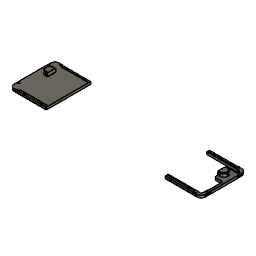
Pianista_podpera_klasvesy (Autodesk Fusion 360 design; units mm, degrees)
Autodesk Fusion 360 part; units mm, degrees
note: some values were not read from the file. Chosen so that the rebuilt part matches the saved one: which face or edge a step refers to. Set by a fixed rule: which sketch regions a step uses.
sketch "Sketch1" plane through (0, 0, 0) normal (0, 0, 1) x (1, 0, 0)
  line L0 (0, 0) -> (-465, 0)
  line L1 (-465, 0) -> (-465, 250)
  line L2 (-465, 250) -> (0, 250)
  line L3 (-275, 250) -> (-275, 0)
  line L4 (0, 0) -> (465, 0)
  line L5 (465, 0) -> (465, 250)
  line L6 (275, 250) -> (275, 0)
  line L7 (465, 250) -> (0, 250)
  line L8 (0, 0) -> (0, 110)
  line L9 (-443, 13) -> (-443, 222)
  line L10 (-443, 222) -> (0, 222)
  line L11 (443, 13) -> (443, 222)
  line L12 (443, 222) -> (0, 222)
  line L13 (0, 13) -> (443, 13)
  line L14 (0, 13) -> (-443, 13)
  line L15 (-465, 250) -> (-465, 176.5)
  line L16 (-465, 0) -> (-465, 145.5)
  line L17 (-422.875, 157.5) -> (-422.875, 176.5)
  line L18 (-423, 157.5) -> (-423, 138.5)
  line L19 (-465, 0) -> (-438, 0)
  circle A0 centre (-438, 45) radius 3
  circle A1 centre (438, 45) radius 3
  circle A2 centre (-438, 45) radius 1.8
  circle A3 centre (438, 45) radius 1.8
  line L20 (0, 28) -> (-425, 28)
  line L21 (-423, 207) -> (0, 207)
  line L22 (-398.9602, 123.8181) -> (-428.0977, 123.2487)
  line L23 (-394.0579, 128.8187) -> (-394.075, 186.5015)
  line L24 (-399.075, 191.5) -> (-428, 191.5)
  line L25 (-430, 33) -> (-430, 55)
  line L26 (-433, 57) -> (-433, 118.2497)
  arc A4 (-423, 207) -> (-433, 197) centre (-423, 197) ccw
  arc A5 (-430, 33) -> (-425, 28) centre (-425, 33) ccw
  arc A6 (-394.075, 186.5015) -> (-399.075, 191.5) centre (-399.075, 186.5) ccw
  arc A7 (-398.9602, 123.8181) -> (-394.0579, 128.8187) centre (-399.0579, 128.8172) ccw
  arc A8 (-428.0977, 123.2487) -> (-433, 118.2497) centre (-428, 118.2497) ccw
  line L27 (-433, 197) -> (-433, 196.5)
  arc A9 (-433, 196.5) -> (-428, 191.5) centre (-428, 196.5) ccw
  line L28 (-404.0722, 177) -> (-275, 177)
  line L29 (-404.075, 138.4) -> (-275, 138.4)
  line L30 (423, 207) -> (0, 207)
  arc A10 (433, 197) -> (423, 207) centre (423, 197) ccw
  line L31 (433, 197) -> (433, 196.5)
  arc A11 (428, 191.5) -> (433, 196.5) centre (428, 196.5) ccw
  line L32 (399.075, 191.5) -> (428, 191.5)
  line L33 (404.0722, 177) -> (275, 177)
  line L34 (404.075, 138.4) -> (275, 138.4)
  line L35 (394.0579, 128.8187) -> (394.075, 186.5015)
  arc A12 (399.075, 191.5) -> (394.075, 186.5015) centre (399.075, 186.5) ccw
  line L36 (-432, 56) -> (-431, 56)
  arc A13 (-433, 57) -> (-432, 56) centre (-432, 57) ccw
  arc A14 (-430, 55) -> (-431, 56) centre (-431, 55) ccw
  arc A15 (394.0579, 128.8187) -> (398.9602, 123.8181) centre (399.0579, 128.8172) ccw
  line L37 (398.9602, 123.8181) -> (428.0977, 123.2487)
  arc A16 (433, 118.2497) -> (428.0977, 123.2487) centre (428, 118.2497) ccw
  line L38 (433, 57) -> (433, 118.2497)
  arc A17 (432, 56) -> (433, 57) centre (432, 57) ccw
  line L39 (432, 56) -> (431, 56)
  arc A18 (431, 56) -> (430, 55) centre (431, 55) ccw
  line L40 (430, 33) -> (430, 55)
  arc A19 (425, 28) -> (430, 33) centre (425, 33) ccw
  line L41 (0, 28) -> (425, 28)
  arc A20 (-404.0722, 177) -> (-404.075, 138.4) centre (-403.6974, 157.7) ccw
  arc A21 (404.075, 138.4) -> (404.0722, 177) centre (403.6974, 157.7) ccw
  point P0 (-394.0765, 191.5)
  dimension "d1" = 465
  dimension "d2" = 250
  dimension "d33" = 550
  dimension "d96" = 73.5
  dimension "d97" = 145.5
  dimension "d104" = 19
  dimension "d105" = 42
  dimension "d114" = 27
  dimension "d115" = 45
  dimension "d116" = 6
  dimension "d120" = 3.6
  dimension "d127" = 15
  dimension "d128" = 15
  dimension "d129" = 10
  dimension "d131" = 5
  dimension "d132" = 5
  dimension "d133" = 5
  dimension "d134" = 5
  dimension "d135" = 5
  dimension "d138" = 10
  dimension "d139" = 14.5
  dimension "d144" = 38.6
  dimension "d145" = 1
  dimension "d146" = 1
  constraint coincident L0.start L4.start
  constraint perpendicular L0 L8
  constraint perpendicular L0 L1
  constraint perpendicular L0 L3
  constraint symmetric L0.start L4.start L8
  constraint symmetric L0.end L4.end L8
  constraint symmetric L1.end L5.end L8
  constraint coincident L2 L3.start
  constraint coincident L0 L3.end
  constraint perpendicular L2 L15
  constraint perpendicular L0 L16
  constraint perpendicular L16 L19
  constraint symmetric L8 A0 A1
  constraint concentric A0 A2
  constraint symmetric L8 A2 A3
  constraint perpendicular L9 L24
  constraint coincident P0 L23
  constraint tangent L21 A4
  constraint tangent L26 A4
  constraint tangent L25 A5
  constraint tangent L20 A5
  constraint coincident P0 L24
  constraint tangent L24 A6
  constraint tangent L23 A6
  constraint tangent L22 A7
  constraint tangent L23 A7
  constraint coincident L26 A4.end
  constraint tangent L26 A8
  constraint tangent L22 A8
  constraint tangent A4 L27
  constraint perpendicular L24 L27
  constraint tangent L27 A9
  constraint tangent L24 A9
  constraint coincident L18.start A20
  constraint symmetric L8 L21.end L30.end
  constraint symmetric L8 L21.start L30.start
  constraint symmetric L8 A4.end A10.start
  constraint symmetric L8 A4 A10
  constraint symmetric L8 L24.start L32.start
  constraint symmetric L8 L23.end L35.end
  constraint symmetric L8 A6 A12
  constraint symmetric L8 L23.start L35.start
  constraint symmetric L8 L27.end L31.end
  constraint symmetric L8 L24.end A11.start
  constraint symmetric L8 A9 A11
  constraint symmetric L8 L28.start L33.start
  constraint symmetric L8 L28.end L33.end
  constraint symmetric L8 L29.start L34.start
  constraint symmetric L8 L29.end L34.end
  constraint symmetric L8 A20 A21
  constraint perpendicular L25 L36
  constraint tangent L26 A13
  constraint tangent L36 A13
  constraint tangent L36 A14
  constraint tangent L25 A14
  constraint symmetric L8 L20.start L41.start
  constraint symmetric L8 L25.start L40.start
  constraint symmetric L8 L20.end A19.start
  constraint symmetric L8 A5 A19
  constraint symmetric L8 L22.start A15.end
  constraint symmetric L8 A7 A15
  constraint symmetric L8 L26.end A16.start
  constraint symmetric L8 L22.end L37.end
  constraint symmetric L8 A8 A16
  constraint symmetric L8 L26.start L38.start
  constraint symmetric L8 L36.start A17.start
  constraint symmetric L8 A13 A17
  constraint symmetric L8 L36.end L39.end
  constraint symmetric L8 L25.end A18.end
  constraint symmetric L8 A14 A18
  measures "d1" distance of L0.start L0.end
  measures "d2" distance of L0.start L2.end
  measures "d33" distance of L3.end L6.end
  measures "d96" distance of L1.end L15.end
  measures "d97" distance of L0.end L16.end
  measures "d104" distance of L17.start L17.end
  measures "d105" distance of L1 L18.start
  measures "d114" distance of L0.end L19.end
  measures "d115" distance of L19.end A0.centre
  measures "d116" diameter of A0
  measures "d120" diameter of A2
  measures "d127" distance of L10 L21
  measures "d128" distance of L14 L20
  measures "d129" radius of A4
  measures "d131" radius of A5
  measures "d132" radius of A6
  measures "d133" radius of A7
  measures "d134" radius of A8
  measures "d135" radius of A9
  measures "d138" distance of L23 L28.start
  measures "d139" distance of L24 L28.start
  measures "d144" distance of L28 L29
  measures "d145" radius of A13
  measures "d146" radius of A14
extrude "Extrude1" add sketch "Sketch1" along normal blind 11.5 contours L3 L9 L10 L14 L20 L21 L22 L23 L24 L25 L26 A4 A5 A6 A7 A8 L27 A9 L28 L29 L36 A13 A14 A20 | L6 L11 L12 L13 L30 A10 L31 A11 L32 L33 L34 L35 A12 A15 L37 A16 L38 A17 L39 A18 L40 A19 L41 A21 | L3 L20 L22 L23 L25 L26 A5 A7 A8 L29 L36 A13 A14 | L3 L23 L28 L29 | L3 L21 L23 L24 A4 A6 L27 A9 L28 | L23 L28 L29 A20 | L33 L34 L35 A21 | A0 | A1 | A2 | A3 makes body 1 at (416.7185, 147.8558, 0) makes body 2 at (-387, 152.3333, 0)
fillet "Fillet2" radius 20 4 edges at (443, 13, 5.75) (443, 222, 5.75) (-443, 13, 5.75) (-443, 222, 5.75) on bodies 1 2
sketch "Sketch3" plane through (443, 0, 0) normal (1, 0, 0) x (0, 1, 0)
  line L0 (13, 0) -> (222, 0)
  line L1 (117.5, 0) -> (117.5, 10)
  line L2 (202, 0) -> (202, 11.5)
  line L3 (202, 11.5) -> (183.5, 11.5)
  line L4 (183.5, 11.5) -> (183.5, 0)
  line L5 (117.5, 0, -886) -> (117.5, 10, -886)
  line L6 (41, 11.5) -> (59.5, 11.5)
  line L7 (41, 5.75) -> (59.5, 5.75)
  line L8 (41, 0) -> (41, 11.5)
  line L9 (59.5, 11.5) -> (59.5, 0)
  circle A0 centre (50.25, 5.75) radius 1.6
  line L10 (59.5802, 11.5105, -886) -> (59.5802, 0.0105, -886)
  line L11 (41.0802, 11.5105, -886) -> (59.5802, 11.5105, -886)
  line L12 (41.0802, 0.0105, -886) -> (41.0802, 11.5105, -886)
  line L13 (59.5802, 5.7605, -886) -> (41.0802, 5.7605, -886)
  line L14 (202.0003, 0.0105, -886) -> (41.0802, 0.0105, -886)
  line L15 (186.5015, 10, -48.925) -> (128.8187, 10, -48.9421)
  line L16 (157.6601, 10, -48.9336) -> (157.6601, 16.0338, -48.9336)
  line L17 (157.6601, 16.0338, -48.9336) -> (157.6601, 16.0338, -19.9336)
  circle A1 through (159.1094, 16.034, -19.8895) (156.9351, 17.2894, -19.9517) (156.9357, 14.7779, -19.9595)
  line L18 (157.6601, 16.0338, -19.9336) -> (157.6601, 16.0338, 0.0664)
  line L19 (157.6601, 16, -885.9336) -> (157.6601, 16, -865.9336)
  circle A2 through (159.1101, 16, -865.9336) (156.9351, 17.2557, -865.9336) (156.9351, 14.7443, -865.9336)
  line L20 (202, 0) -> (202, 11.5)
  line L21 (202, 11.5) -> (33, 11.5)
  line L22 (33, 11.5) -> (33, 0)
  line L23 (33, 0) -> (202, 0)
  line L24 (13, 11.5) -> (13, 1.2)
  line L25 (13, 11.5) -> (23.3, 11.5)
  line L26 (23.3, 11.5) -> (23.3, 10.35)
  line L27 (13, 1.2) -> (14.15, 1.2)
  line L28 (14.15, 1.2) -> (14.15, 10.35)
  line L29 (14.15, 10.35) -> (23.3, 10.35)
  line L30 (211.7, 11.5) -> (211.7, 10.35)
  line L31 (220.85, 10.35) -> (211.7, 10.35)
  line L32 (220.85, 1.2) -> (220.85, 10.35)
  line L33 (222, 1.2) -> (220.85, 1.2)
  line L34 (222, 11.5) -> (222, 1.2)
  line L35 (222, 11.5) -> (211.7, 11.5)
  line L36 (183.5, 5.75) -> (202, 5.75)
  circle A3 centre (192.75, 5.75) radius 1.6
  line L37 (202, 0) -> (202, 11.5)
  line L38 (183.5, 0) -> (183.5, 11.5)
  line L39 (183.5, 0, -886) -> (183.5, 11.5, -886)
  line L40 (202, 11.5, -886) -> (183.5, 11.5, -886)
  line L41 (183.5, 11.5, -886) -> (183.5, 0, -886)
  circle A4 through (194.35, 5.75, -886) (191.95, 7.1356, -886) (191.95, 4.3644, -886)
  line L42 (183.5, 5.75, -886) -> (202, 5.75, -886)
  line L43 (202, 0, -886) -> (202, 11.5, -886)
  line L44 (202, 0, -886) -> (202, 11.5, -886)
  circle A5 through (51.9302, 5.7605, -886) (49.5302, 7.1462, -886) (49.5302, 4.3749, -886)
  point P0 (33, 10)
  point P1 (202, 10)
  dimension "d157" = 209
  dimension "d186" = 18.5
  dimension "d187" = 11.5
  dimension "d188" = 3.2
  dimension "d189" = 18.5
  dimension "d190" = 11.5
  dimension "d217" = 29
  dimension "d218" = 2.9
  dimension "d221" = 20
  dimension "d223" = 20
  dimension "d224" = 2.9
  dimension "d262" = 10.3
  dimension "d263" = 10.3
  dimension "d264" = 1.15
  dimension "d265" = 1.15
  dimension "d266" = 11.5
  dimension "d267" = 11.5
  dimension "d268" = 3.2
  dimension "d270" = 11.5
  dimension "d271" = 11.5
  dimension "d272" = 3.2
  dimension "d277" = 3.2
  constraint midpoint L0 L1.start
  constraint perpendicular L0 L1
  constraint horizontal L6
  constraint vertical L9
  constraint vertical L8
  constraint midpoint L7.start L8
  constraint midpoint L7.end L9
  constraint midpoint A0.centre L7
  constraint vertical L24
  constraint perpendicular L24 L25
  constraint perpendicular L25 L26
  constraint perpendicular L24 L27
  constraint perpendicular L27 L28
  constraint perpendicular L26 L29
  constraint symmetric L1 L24.start L34.start
  constraint symmetric L1 L24.end L33.start
  constraint symmetric L1 L25.end L30.start
  constraint symmetric L1 L26.end L30.end
  constraint symmetric L1 L27.end L32.start
  constraint symmetric L1 L28.end L31.start
  constraint midpoint L4 L36.start
  constraint midpoint L20 L36.end
  constraint perpendicular L20 L36
  constraint midpoint L36 A3.centre
  constraint coincident L2.end L3.start
  constraint perpendicular L21 L38
  measures "d157" distance of L0.start L0.end
  measures "d186" distance of L6.start L6.end
  measures "d187" distance of L6.start L8.start
  measures "d188" diameter of A0
  measures "d262" distance of L24.start L24.end
  measures "d263" distance of L24.start L25.end
  measures "d264" distance of L25.end L26.end
  measures "d265" distance of L24.end L27.end
  measures "d266" distance of L3.end L4.end
  measures "d267" distance of L2.start L2.end
  measures "d268" diameter of A3
  measures "d270" distance of L3.end L4.end
  measures "d271" distance of L2.end L2.start
extrude "Extrude21" cut sketch "Sketch3" against normal blind 0.7 contours L0 L7 L8 L9 A0 L23 | L6 L7 L8 L9 A0 L21 | L7 A0 | L7 A0 | L0 L2 L4 L20 L23 L36 A3 L37 L38 | L2 L3 L4 L20 L21 L36 A3 L37 L38 | L36 A3 | L36 A3 bodies 1
sketch "Sketch3 (curves -886 mm off its plane)" plane through (-443, 0, 0) normal (1, 0, 0) x (0, 1, 0)
  line L0 (117.5, 0) -> (117.5, 10)
  line L1 (59.5802, 11.5105) -> (59.5802, 0.0105)
  line L2 (41.0802, 11.5105) -> (59.5802, 11.5105)
  line L3 (41.0802, 0.0105) -> (41.0802, 11.5105)
  line L4 (59.5802, 5.7605) -> (41.0802, 5.7605)
  line L5 (202.0003, 0.0105) -> (41.0802, 0.0105)
  line L6 (183.5, 0) -> (183.5, 11.5)
  line L7 (202, 11.5) -> (183.5, 11.5)
  line L8 (183.5, 11.5) -> (183.5, 0)
  circle A0 centre (192.75, 5.75) radius 1.6
  line L9 (183.5, 5.75) -> (202, 5.75)
  line L10 (202, 0) -> (202, 11.5)
  line L11 (202, 0) -> (202, 11.5)
  circle A1 centre (50.3302, 5.7605) radius 1.6
extrude "Extrude22" cut sketch "Sketch3 (curves -886 mm off its plane)" along normal blind 0.7 bodies 2
extrude "Extrude10" add sketch "Sketch1" along normal blind 16 from surface at 11.5 contours L23 L28 L29 A20 | L33 L34 L35 A21 bodies 1 2
fillet "Fillet4" radius 3 6 edges at (399.0722, 177, 27.5) (399.0679, 138.4, 27.5) (423.001, 157.7014, 27.5) (-399.0722, 177, 27.5) (-423.001, 157.7014, 27.5) (-399.0679, 138.4, 27.5) on bodies 1 2
extrude "Extrude12" cut sketch "Sketch1" along normal blind 11.5 contours A2 | A3 bodies 1 2
extrude "Extrude11" cut sketch "Sketch1" against normal blind 6.5 from surface at 11.5 contours A0 | A1 | A2 | A3 bodies 1 2
extrude "Extrude4" cut sketch "Sketch3" against normal blind 809 from surface at -38.5 contours L24 L25 L26 L27 L28 L29 | L30 L31 L32 L33 L34 L35 bodies 1 2
extrude "Extrude13" cut 1 faces at (416.8333, 13, 4.2333) along direction (0, 1, 0) blind 0.7 on bodies 1 bodies 1
extrude "Extrude14" cut 1 faces at (416.8333, 222, 4.2333) along direction (0, -1, 0) blind 0.7 on bodies 1 bodies 1
extrude "Extrude15" cut 1 faces at (-416.8333, 222, 4.2333) along direction (0, -1, 0) blind 0.7 on bodies 2 bodies 2
extrude "Extrude16" cut 1 faces at (-416.8333, 13, 4.2333) along direction (0, 1, 0) blind 0.7 on bodies 2 bodies 2
sketch "Sketch4" plane through (0, 13.7, 0) normal (0, -1, 0) x (1, 0, 0)
  line L0 (275, 0) -> (423, 0)
  line L1 (423, 11.5) -> (404.5, 11.5)
  line L2 (404.0722, 11.5, -163.3) -> (404.0722, 24.5, -163.3)
  line L3 (394.0722, 11.5, -163.3) -> (394.0722, 24.5, -163.3)
  line L4 (404.0722, 18, -163.3) -> (394.0722, 18, -163.3)
  circle A0 through (400.5222, 18, -163.3) (398.3472, 19.2557, -163.3) (398.3472, 16.7443, -163.3)
  line L5 (394.0607, 11.5, -124.7) -> (394.0607, 24.5, -124.7)
  line L6 (404.075, 11.5, -124.7) -> (404.075, 24.5, -124.7)
  line L7 (394.0607, 18, -124.7) -> (404.075, 18, -124.7)
  circle A1 through (400.5179, 18, -124.7) (398.3429, 19.2557, -124.7) (398.3429, 16.7443, -124.7)
  line L8 (-404.075, 11.5, -124.7) -> (-404.075, 24.5, -124.7)
  line L9 (-394.0607, 11.5, -124.7) -> (-394.0607, 24.5, -124.7)
  line L10 (-404.075, 18, -124.7) -> (-394.0607, 18, -124.7)
  circle A2 through (-397.6179, 18, -124.7) (-399.7929, 19.2557, -124.7) (-399.7929, 16.7443, -124.7)
  line L11 (-404.0722, 11.5, -163.3) -> (-404.0722, 24.5, -163.3)
  line L12 (-394.0722, 11.5, -163.3) -> (-394.0722, 24.5, -163.3)
  line L13 (-404.0722, 18, -163.3) -> (-394.0722, 18, -163.3)
  circle A3 through (-397.6222, 18, -163.3) (-399.7972, 19.2557, -163.3) (-399.7972, 16.7443, -163.3)
  line L14 (423, 11.5) -> (423, 0)
  line L15 (423, 0, -207.6) -> (423, 11.5, -207.6)
  line L16 (275, 1.2) -> (275, 0)
  line L17 (404.5, 1.2) -> (275, 1.2)
  line L18 (404.5, 11.5, -207.6) -> (404.5, 0, -207.6)
  line L19 (404.5, 5.75, -207.6) -> (423, 5.75, -207.6)
  circle A4 through (415.35, 5.75, -207.6) (412.95, 7.1356, -207.6) (412.95, 4.3644, -207.6)
  line L20 (404.5, 11.5) -> (404.5, 0)
  line L21 (404.5, 5.75) -> (423, 5.75)
  circle A5 centre (413.75, 5.75) radius 1.6
  line L22 (-404.5, 11.5, -207.6) -> (-404.5, 0, -207.6)
  line L23 (-423, 11.5, -207.6) -> (-423, 0, -207.6)
  line L24 (-404.5, 5.75, -207.6) -> (-423, 5.75, -207.6)
  circle A6 through (-412.15, 5.75, -207.6) (-414.55, 7.1356, -207.6) (-414.55, 4.3644, -207.6)
  line L25 (-404.5, 11.5) -> (-404.5, 0)
  line L26 (-423, 11.5) -> (-423, 0)
  line L27 (-423, 5.75) -> (-404.5, 5.75)
  circle A7 centre (-413.75, 5.75) radius 1.6
  point P0 (404.5, 11.5)
  point P1 (-404.5, 11.5)
  point P2 (-423, 11.5)
  point P3 (-423, 0)
  point P4 (-404.5, 11.5)
  point P5 (-423, 11.5)
  point P6 (-423, 0)
  dimension "d208" = 2.9
  dimension "d209" = 2.9
  dimension "d210" = 2.9
  dimension "d211" = 2.9
  dimension "d273" = 3.2
  dimension "d274" = 3.2
  dimension "d275" = 3.2
  dimension "d276" = 3.2
  constraint coincident P0 L1.end
  constraint coincident L0 L20.end
  constraint perpendicular L0 L20
  constraint midpoint L20 L21.start
  constraint perpendicular L20 L21
  constraint midpoint L21 A5.centre
  constraint coincident P4 P1
  constraint coincident P5 P2
  constraint coincident P6 P3
  constraint midpoint L26 L27.start
  constraint midpoint L25 L27.end
  constraint midpoint L27 A7.centre
  measures "d274" diameter of A5
  measures "d276" diameter of A7
sketch "Sketch4 (curves -207.6 mm off its plane)" plane through (0, 221.3, 0) normal (0, -1, 0) x (1, 0, 0)
  line L0 (423, 0) -> (423, 11.5)
  line L1 (404.5, 11.5) -> (404.5, 0)
  line L2 (404.5, 5.75) -> (423, 5.75)
  circle A0 centre (413.75, 5.75) radius 1.6
  line L3 (-404.5, 11.5) -> (-404.5, 0)
  line L4 (-423, 11.5) -> (-423, 0)
  line L5 (-404.5, 5.75) -> (-423, 5.75)
  circle A1 centre (-413.75, 5.75) radius 1.6
extrude "Extrude17" cut sketch "Sketch4 (curves -207.6 mm off its plane)" along normal blind 12 bodies 1 2
extrude "Extrude18" cut sketch "Sketch4" against normal blind 12 contours L21 A5 | L21 A5 | L27 A7 | L27 A7 bodies 1 2
extrude "Extrude19" cut sketch "Sketch3 (curves -886 mm off its plane)" along normal blind 12 from surface at 0.7 contours L4 A1 | L4 A1 | A0 L9 | A0 L9 bodies 2
extrude "Extrude20" cut sketch "Sketch3" against normal blind 12 from surface at -0.7 contours L7 A0 | L7 A0 | L36 A3 | L36 A3 bodies 1
sketch "Sketch5" plane through (0, 0, 10.35) normal (0, 0, 1) x (-1, 0, 0)
  line L0 (275, -211.7) -> (275, -220.85)
  line L1 (275, -220.85) -> (404.5, -220.85)
  line L2 (404.5, -220.85) -> (404.5, -211.7)
  line L3 (404.5, -211.7) -> (275, -211.7)
  line L4 (404.5, -211.7) -> (404.5, -220.85)
  line L5 (404.5, -216.275) -> (275, -216.275)
  line L6 (339.75, -216.275) -> (379.75, -216.275)
  line L7 (339.75, -216.275) -> (299.75, -216.275)
  circle A0 centre (299.75, -216.275) radius 1.6
  circle A1 centre (379.75, -216.275) radius 1.6
  line L8 (404.5, -14.15) -> (404.5, -23.3)
  line L9 (404.5, -18.725) -> (275, -18.725)
  circle A2 centre (379.75, -18.725) radius 1.6
  circle A3 centre (299.75, -18.725) radius 1.6
  line L10 (-275, -14.15) -> (-275, -23.3)
  line L11 (-275, -18.725) -> (-404.5, -18.725)
  circle A4 centre (-299.75, -18.725) radius 1.6
  circle A5 centre (-379.75, -18.725) radius 1.6
  line L12 (-275, -211.7) -> (-275, -220.85)
  line L13 (-275, -216.275) -> (-404.5, -216.275)
  circle A6 centre (-299.75, -216.275) radius 1.6
  circle A7 centre (-379.75, -216.275) radius 1.6
  circle A8 centre (438, -45) radius 1.8
  line L14 (275, -211.7) -> (275, -220.85)
  line L15 (275, -220.85) -> (404.5, -220.85)
  line L16 (404.5, -220.85) -> (404.5, -211.7)
  line L17 (404.5, -211.7) -> (275, -211.7)
  point P0 (-379.75, -216.275)
  dimension "d196" = 40
  dimension "d197" = 40
  dimension "d198" = 3.2
  dimension "d199" = 3.2
  dimension "d200" = 3.2
  dimension "d201" = 3.2
  dimension "d202" = 3.2
  dimension "d203" = 3.2
  dimension "d204" = 3.2
  dimension "d207" = 3.2
  constraint coincident L2.end L3.start
  constraint coincident L1.end L2.start
  constraint midpoint L2 L5.start
  constraint perpendicular L2 L5
  constraint coincident L0 L5.end
  constraint midpoint L5 L6.start
  constraint parallel L5 L6
  constraint parallel L5 L7
  constraint coincident L7.end A0.centre
  constraint coincident L6.end A1.centre
  constraint coincident P0 A7.centre
  measures "d196" distance of L6.start L6.end
  measures "d197" distance of L6.start L7.end
  measures "d198" diameter of A0
  measures "d199" diameter of A1
  measures "d200" diameter of A3
  measures "d201" diameter of A2
  measures "d202" diameter of A6
  measures "d203" diameter of A5
  measures "d204" diameter of A4
  measures "d207" diameter of A7
extrude "Extrude23" cut sketch "Sketch5" against normal blind 10.35 contours L5 L7 A0 | L5 L7 A0 | L5 L6 A1 | L5 L6 A1 | L9 A2 | L9 A2 | L9 A3 | L9 A3 | L11 A4 | L11 A4 | L11 A5 | L11 A5 | L13 A6 | L13 A6 | L13 A7 | L13 A7 bodies 1 2
sketch "Sketch4 (curves -163.3 mm off its plane)" plane through (0, 177, 0) normal (0, -1, 0) x (1, 0, 0)
  line L0 (404.0722, 11.5) -> (404.0722, 24.5)
  line L1 (394.0722, 11.5) -> (394.0722, 24.5)
  line L2 (404.0722, 18) -> (394.0722, 18)
  circle A0 centre (399.0722, 18) radius 1.45
  line L3 (-404.0722, 11.5) -> (-404.0722, 24.5)
  line L4 (-394.0722, 11.5) -> (-394.0722, 24.5)
  line L5 (-404.0722, 18) -> (-394.0722, 18)
  circle A1 centre (-399.0722, 18) radius 1.45
extrude "Extrude24" cut sketch "Sketch4 (curves -163.3 mm off its plane)" along normal blind 12 bodies 1 2
sketch "Sketch4 (curves -124.7 mm off its plane)" plane through (0, 138.4, 0) normal (0, -1, 0) x (1, 0, 0)
  line L0 (394.0607, 11.5) -> (394.0607, 24.5)
  line L1 (404.075, 11.5) -> (404.075, 24.5)
  line L2 (394.0607, 18) -> (404.075, 18)
  circle A0 centre (399.0679, 18) radius 1.45
  line L3 (-404.075, 11.5) -> (-404.075, 24.5)
  line L4 (-394.0607, 11.5) -> (-394.0607, 24.5)
  line L5 (-404.075, 18) -> (-394.0607, 18)
  circle A1 centre (-399.0679, 18) radius 1.45
extrude "Extrude25" cut sketch "Sketch4 (curves -124.7 mm off its plane)" against normal blind 12 bodies 1 2
sketch "Sketch3 (curves on the plane with normal 0.9995, -0.0304, -0.0031 at -24.7642 mm)" plane through (418.2473, 0.7524, 0.0772) normal (0.999534, -0.030381, -0.003119) x (0, 0.102131, -0.994771)
  circle A0 centre (0.152, 157.7905) radius 1.45
extrude "Extrude26" cut sketch "Sketch3 (curves on the plane with normal 0.9995, -0.0304, -0.0031 at -24.7642 mm)" against normal blind 12 bodies 1
sketch "Sketch3 (curves -865.9336 mm off its plane)" plane through (-422.9336, 0, 0) normal (1, 0, 0) x (0, 1, 0)
  circle A0 centre (157.6601, 16) radius 1.45
extrude "Extrude27" cut sketch "Sketch3 (curves -865.9336 mm off its plane)" along normal blind 12 from surface at -0.1 bodies 2
chamfer "Chamfer1" distance 2 angle 45 22 edges at (397.716, 138.4, 18.5243) (397.7203, 177, 17.4757) (442.3, 48.7583, 6.3286) (381.2417, 18.1464, 10.35) (301.2417, 18.1464, 10.35) (301.2417, 215.6964, 10.35) (381.2417, 215.6964, 10.35) (422.9492, 159.1143, 16.0341) (412.2583, 13.7, 6.3286) (442.3, 191.2583, 6.3286) (412.2583, 221.3, 5.1714) (-400.4197, 138.4, 18.5243) (-400.4241, 177, 17.4757) (-378.2583, 18.1464, 10.35) (-298.2583, 18.1464, 10.35) (-378.2583, 215.6964, 10.35) (-298.2583, 215.6964, 10.35) (-422.9435, 156.2101, 16) (-415.2417, 221.3, 5.1714) (-415.2417, 13.7, 6.3286) (-442.3, 191.2583, 5.1714) (-442.3, 48.8385, 5.1819) on bodies 1 2
sketch "Sketch6" plane through (0, 0, 0) normal (0, 0, 1) x (1, 0, 0)
  line L0 (298.25, -33.6768) -> (296.75, -36.2749)
  line L1 (301.25, -33.6768) -> (298.25, -33.6768)
  line L2 (298.25, -38.873) -> (301.25, -38.873)
  line L3 (302.75, -36.2749) -> (301.25, -33.6768)
  line L4 (301.25, -38.873) -> (302.75, -36.2749)
  line L5 (296.75, -36.2749) -> (298.25, -38.873)
  line L6 (0, 0) -> (0, 110)
  line L7 (-298.1923, 21.4232) -> (-296.6345, 18.7251)
  line L8 (-302.8655, 18.7251) -> (-301.3077, 21.4232)
  line L9 (-382.8655, 18.7251) -> (-381.3077, 21.4232)
  line L10 (-378.1923, 16.027) -> (-381.3077, 16.027)
  line L11 (-378.1923, 21.4232) -> (-376.6345, 18.7251)
  line L12 (-296.6345, 18.7251) -> (-298.1923, 16.027)
  line L13 (-381.3077, 16.027) -> (-382.8655, 18.7251)
  line L14 (-376.6345, 18.7251) -> (-378.1923, 16.027)
  line L15 (-301.3077, 16.027) -> (-302.8655, 18.7251)
  line L16 (-381.3077, 21.4232) -> (-378.1923, 21.4232)
  line L17 (-302.8655, 216.2751) -> (-301.3077, 218.9732)
  line L18 (-376.6345, 216.2751) -> (-378.1923, 213.577)
  line L19 (-301.3077, 218.9732) -> (-298.1923, 218.9732)
  line L20 (-378.1923, 218.9732) -> (-376.6345, 216.2751)
  line L21 (-381.3077, 213.577) -> (-382.8655, 216.2751)
  line L22 (-381.3077, 218.9732) -> (-378.1923, 218.9732)
  line L23 (-301.3077, 213.577) -> (-302.8655, 216.2751)
  line L24 (-298.1923, 218.9732) -> (-296.6345, 216.2751)
  line L25 (-301.3077, 21.4232) -> (-298.1923, 21.4232)
  line L26 (-378.1923, 213.577) -> (-381.3077, 213.577)
  line L27 (-298.1923, 16.027) -> (-301.3077, 16.027)
  line L28 (-298.1923, 213.577) -> (-301.3077, 213.577)
  line L29 (-296.6345, 216.2751) -> (-298.1923, 213.577)
  line L30 (-382.8655, 216.2751) -> (-381.3077, 218.9732)
  line L31 (-275, 13.7) -> (-423, 13.7)
  line L32 (-423, 221.3) -> (-275, 221.3)
  line L33 (-416.6, 214.3) -> (-410.9, 214.3)
  line L34 (-416.6, 217.3) -> (-416.6, 214.3)
  line L35 (-410.9, 214.3) -> (-410.9, 217.3)
  line L36 (-416.6, 217.3) -> (-410.9, 214.3) construction
  line L37 (-410.9, 217.3) -> (-416.6, 217.3)
  line L38 (-410.9, 217.3) -> (-416.6, 214.3) construction
  line L39 (442.3, 202) -> (442.3, 183.5)
  line L40 (-443, 183.5, 0.0105) -> (-443, 202, 0.0105)
  line L41 (442.3, 192.75, 0) -> (-443, 192.75, 0.0105)
  line L42 (-438.3, 189.95) -> (-435.3, 189.95)
  line L43 (-435.3, 195.65) -> (-438.3, 195.65)
  line L44 (-438.3, 195.65) -> (-435.3, 189.95) construction
  line L45 (-438.3, 189.95) -> (-435.3, 195.65) construction
  line L46 (-438.3, 195.65) -> (-438.3, 189.95)
  line L47 (-435.3, 189.95) -> (-435.3, 195.65)
  line L48 (-442.3, 183.5) -> (-442.3, 202)
  line L49 (435.3, 189.95) -> (438.3, 189.95)
  line L50 (435.3, 189.95) -> (438.3, 195.65) construction
  line L51 (438.3, 189.95) -> (438.3, 195.65)
  line L52 (435.3, 195.65) -> (435.3, 189.95)
  line L53 (438.3, 195.65) -> (435.3, 195.65)
  line L54 (435.3, 195.65) -> (438.3, 189.95) construction
  line L55 (-435, 53.15) -> (-432, 47.45) construction
  line L56 (-435, 47.45) -> (-432, 53.15) construction
  line L57 (-432, 47.45) -> (-432, 53.15)
  line L58 (-435, 47.45) -> (-432, 47.45)
  line L59 (-435, 53.15) -> (-435, 47.45)
  line L60 (-432, 53.15) -> (-435, 53.15)
  line L61 (442.3, 50.25, 0) -> (-443, 50.2428, 0.0105)
  line L62 (434.3, 47.2216) -> (434.3, 52.9216)
  line L63 (434.3, 52.9216) -> (431.3, 52.9216)
  line L64 (431.3, 52.9216) -> (431.3, 47.2216)
  line L65 (431.3, 47.2216) -> (434.3, 52.9216) construction
  line L66 (431.3, 47.2216) -> (434.3, 47.2216)
  line L67 (442.3, 59.5) -> (442.3, 41)
  line L68 (-443, 13) -> (-443, 222)
  line L69 (-413.75, 221.3) -> (-413.75, 13.7)
  line L70 (-410.9, 20.7) -> (-416.6, 20.7)
  line L71 (-416.6, 20.7) -> (-416.6, 17.7)
  line L72 (-416.6, 17.7) -> (-410.9, 17.7)
  line L73 (-410.9, 17.7) -> (-410.9, 20.7)
  line L74 (-410.9, 20.7) -> (-416.6, 17.7) construction
  line L75 (-416.6, 20.7) -> (-410.9, 17.7) construction
  line L76 (-423, 13.7) -> (-404.5, 13.7)
  line L77 (416.6, 217.3) -> (410.9, 214.3) construction
  line L78 (416.6, 217.3) -> (410.9, 217.3)
  line L79 (416.6, 214.3) -> (416.6, 217.3)
  line L80 (410.9, 217.3) -> (410.9, 214.3)
  line L81 (410.9, 214.3) -> (416.6, 214.3)
  line L82 (410.9, 217.3) -> (416.6, 214.3) construction
  line L83 (413.75, 221.3) -> (413.75, 13.7)
  line L84 (410.9, 17.7) -> (416.6, 17.7)
  line L85 (416.6, 20.7) -> (410.9, 20.7)
  line L86 (410.9, 20.7) -> (410.9, 17.7)
  line L87 (416.6, 17.7) -> (416.6, 20.7)
  line L88 (381.3077, 21.4232) -> (378.1923, 21.4232)
  line L89 (376.6345, 216.2751) -> (378.1923, 213.577)
  line L90 (302.8655, 216.2751) -> (301.3077, 218.9732)
  line L91 (296.6345, 18.7251) -> (298.1923, 16.027)
  line L92 (298.1923, 21.4232) -> (296.6345, 18.7251)
  line L93 (298.1923, 16.027) -> (301.3077, 16.027)
  line L94 (298.1923, 218.9732) -> (296.6345, 216.2751)
  line L95 (301.3077, 16.027) -> (302.8655, 18.7251)
  line L96 (302.8655, 18.7251) -> (301.3077, 21.4232)
  line L97 (381.3077, 213.577) -> (382.8655, 216.2751)
  line L98 (378.1923, 16.027) -> (381.3077, 16.027)
  line L99 (381.3077, 16.027) -> (382.8655, 18.7251)
  line L100 (301.3077, 21.4232) -> (298.1923, 21.4232)
  line L101 (382.8655, 216.2751) -> (381.3077, 218.9732)
  line L102 (382.8655, 18.7251) -> (381.3077, 21.4232)
  line L103 (376.6345, 18.7251) -> (378.1923, 16.027)
  line L104 (301.3077, 213.577) -> (302.8655, 216.2751)
  line L105 (381.3077, 218.9732) -> (378.1923, 218.9732)
  line L106 (298.1923, 213.577) -> (301.3077, 213.577)
  line L107 (378.1923, 21.4232) -> (376.6345, 18.7251)
  line L108 (296.6345, 216.2751) -> (298.1923, 213.577)
  line L109 (301.3077, 218.9732) -> (298.1923, 218.9732)
  line L110 (378.1923, 213.577) -> (381.3077, 213.577)
  line L111 (378.1923, 218.9732) -> (376.6345, 216.2751)
  point P0 (299.75, -36.2749)
  point P1 (438, 45.0001)
  point P2 (-379.75, 18.7251)
  point P3 (-379.75, 216.2751)
  point P4 (-438, 45.0001)
  point P5 (-299.75, 216.2751)
  point P6 (-299.75, 18.7251)
  point P7 (-413.75, 215.8)
  point P8 (-436.8, 192.8)
  point P9 (436.8, 192.8)
  point P10 (-433.5, 50.3)
  point P11 (-413.75, 221.3)
  point P12 (-413.75, 19.2)
  point P13 (413.75, 215.8)
  point P14 (299.75, 18.7251)
  point P15 (379.75, 18.7251)
  point P16 (379.75, 216.2751)
  point P17 (299.75, 216.2751)
  dimension "d241" = 5.7
  dimension "d242" = 3
  dimension "d246" = 5.7
  dimension "d247" = 3
  dimension "d248" = 4
  dimension "d249" = 5.7
  dimension "d250" = 3
  dimension "d251" = 4
  dimension "d252" = 5.7
  dimension "d253" = 3
  dimension "d254" = 5.7
  dimension "d255" = 3
  dimension "d256" = 8
  dimension "d257" = 8
  dimension "d281" = 5.7
  dimension "d282" = 3
  dimension "d283" = 4
  dimension "d284" = 4
  dimension "d285" = 5.7
  dimension "d286" = 3
  dimension "d287" = 5.7
  dimension "d288" = 3
  constraint symmetric P1 L6 P4
  constraint horizontal L37
  constraint perpendicular L34 L37
  constraint parallel L33 L37
  constraint parallel L34 L35
  constraint coincident P7 L38
  constraint coincident P7 L36
  constraint perpendicular L42 L46
  constraint parallel L46 L47
  constraint parallel L42 L43
  constraint coincident P8 L44
  constraint coincident P8 L45
  constraint perpendicular L49 L52
  constraint parallel L51 L52
  constraint parallel L49 L53
  constraint coincident P9 L54
  constraint coincident P9 L50
  constraint perpendicular L58 L59
  constraint parallel L57 L59
  constraint parallel L58 L60
  constraint coincident P10 L55
  constraint coincident P10 L56
  constraint perpendicular L64 L66
  constraint parallel L62 L64
  constraint parallel L63 L66
  constraint coincident L32 P11
  constraint coincident L31 L69.end
  constraint perpendicular L31 L69
  constraint horizontal L70
  constraint perpendicular L70 L71
  constraint parallel L70 L72
  constraint parallel L71 L73
  constraint coincident L74 P12
  constraint coincident L75 P12
  constraint coincident L69 P12
  constraint horizontal L78
  constraint perpendicular L78 L80
  constraint parallel L78 L81
  constraint parallel L79 L80
  constraint coincident P13 L77
  constraint coincident P13 L82
  constraint horizontal L85
  constraint perpendicular L85 L86
  constraint parallel L84 L85
  constraint parallel L86 L87
  constraint symmetric L6 P2 P15
  constraint symmetric L6 L18.start L89.start
  constraint symmetric L6 L11.end L103.start
  constraint symmetric L6 P3 P16
  constraint symmetric L6 L10.end L98.end
  constraint symmetric L6 L10.start L98.start
  constraint symmetric L6 L18.end L89.end
  constraint symmetric L6 L21.end L97.end
  constraint symmetric L6 L11.start L88.end
  constraint symmetric L6 L9.end L88.start
  constraint symmetric L6 L9.start L99.end
  constraint symmetric L6 L21.start L97.start
  constraint symmetric L6 L7.start L92.start
  constraint symmetric L6 L22.start L101.end
  constraint symmetric L6 P5 P17
  constraint symmetric L6 L20.start L105.end
  constraint symmetric L6 L7.end L91.start
  constraint symmetric L6 L8.start L95.end
  constraint symmetric L6 P6 P14
  constraint symmetric L6 L23.start L104.start
  constraint symmetric L6 L15.start L93.end
  constraint symmetric L6 L8.end L96.end
  constraint symmetric L6 L19.end L94.start
  constraint symmetric L6 L28.start L106.start
  constraint symmetric L6 L17.end L90.end
  constraint symmetric L6 L17.start L90.start
  constraint symmetric L6 L24.end L94.end
  constraint symmetric L6 L12.end L91.end
  measures "d241" distance of L33.start L33.end
  measures "d242" distance of L34.start L33.start
  measures "d246" distance of L42.end L43.start
  measures "d247" distance of L42.start L42.end
  measures "d248" distance of L46 L48
  measures "d249" distance of L49.end L50.end
  measures "d250" distance of L49.start L49.end
  measures "d251" distance of L39 L51
  measures "d252" distance of L55.end L56.end
  measures "d253" distance of L56.start L55.end
  measures "d254" distance of L62.start L62.end
  measures "d255" distance of L62.start L64.end
  measures "d256" distance of L62 L67
  measures "d257" distance of L59 L68
  measures "d281" distance of L71.end L72.end
  measures "d282" distance of L70.end L71.end
  measures "d283" distance of L72 L76
  measures "d284" distance of L32 L37
  measures "d285" distance of L79.start L77.end
  measures "d286" distance of L78.end L77.end
  measures "d287" distance of L84.end L84.start
  measures "d288" distance of L85.end L84.start
extrude "Extrude30" cut sketch "Sketch6" along normal blind 5 contours L7 L8 L12 L15 L25 L27 | L9 L10 L11 L13 L14 L16 | L17 L19 L23 L24 L28 L29 | L18 L20 L21 L22 L26 L30 | L88 L98 L99 L102 L103 L107 | L89 L97 L101 L105 L110 L111 | L90 L94 L104 L106 L108 L109 | L91 L92 L93 L95 L96 L100 bodies 1 2
extrude "Extrude29" cut sketch "Sketch6" along normal blind 9 contours L33 L34 L37 L69 | L33 L35 L37 L69 | L42 L43 L46 L47 | L49 L51 L52 L53 | L57 L58 L59 L60 | L62 L63 L64 L66 | L69 L70 L72 L73 | L69 L70 L71 L72 | L78 L79 L81 L83 | L78 L80 L81 L83 | L83 L84 L85 L87 | L83 L84 L85 L86 bodies 1 2
equation "tloustka = 2 mm"
named bodies: "Right", "Left"
